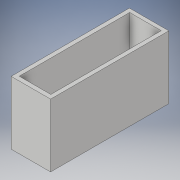
# Autodesk Inventor part: storebox2
Saved by Autodesk Inventor 2019 (Build 230136000, 136)
## iProperties
Created: 2019-10-16
Part Number: storebox2
Material: Generic
Document SubType Name: Modeling
Designer: savan
Density: 1 g/cm^3
Appearance: Default
Author: savan
Autodesk Inventor part; units mm, degrees
ref_plane "YZ Plane" through (0, 0, 0) normal (1, 0, 0) x (0, 1, 0)
ref_plane "XZ Plane" through (0, 0, 0) normal (0, 1, 0) x (-1, 0, 0)
ref_plane "XY Plane" through (0, 0, 0) normal (0, 0, 1) x (1, 0, 0)
sketch "Sketch1" plane through (0, 0, 0) normal (0, 1, 0) x (-1, 0, 0)
  line L0 (0, 0) -> (50, 0)
  line L1 (50, 0) -> (50, -300)
  line L2 (50, -300) -> (0, -300)
  line L3 (0, -300) -> (0, 0)
  dimension "d0" = 50
  dimension "d1" = 300
  constraints: 8 end point, 2 parallel, 1 horizontal, 1 perpendicular
  measures "d0" distance of L1.end L2.end
  measures "d1" distance of L0.end L1.end
extrude "Extrusion1" add sketch "Sketch1" along normal blind 80
sketch "Sketch2" plane through (0, 80, 0) normal (0, 1, 0) x (1, 0, 0)
  line L0 (0, 0) -> (-50, 0)
  line L1 (-50, 0) -> (-50, 150)
  line L2 (-50, 150) -> (0, 150)
  line L3 (0, 150) -> (0, 0)
  dimension "d4" = 50
  dimension "d5" = 150
  constraints: 8 end point, 2 parallel, 1 horizontal, 1 perpendicular
  measures "d4" distance of L1.end L2.end
  measures "d5" distance of L0.end L1.end
extrude "Extrusion2" cut sketch "Sketch2" against normal blind 100
sketch "Sketch3" plane through (0, 80, 0) normal (0, 1, 0) x (1, 0, 0)
  line L0 (-44.983, 155.2795) -> (-4.983, 155.2795)
  line L1 (-4.983, 155.2795) -> (-4.983, 295.2795)
  line L2 (-4.983, 295.2795) -> (-44.983, 295.2795)
  line L3 (-44.983, 295.2795) -> (-44.983, 155.2795)
  point P0 (0, 0)
  dimension "d8" = 40
  dimension "d9" = 140
  constraints: 8 end point, 2 parallel, 1 horizontal, 1 perpendicular
  measures "d8" distance of L2.end L1.end
  measures "d9" distance of L1.end L0.end
extrude "Extrusion3" cut sketch "Sketch3" against normal blind 70
body "Solid1"
